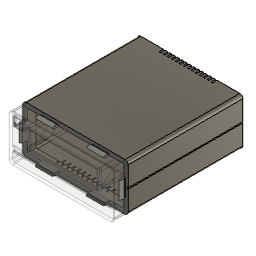
AmigaGotekEnclosure (Autodesk Fusion 360 design; units mm, degrees)
Autodesk Fusion 360 part; units mm, degrees
note: some values were not read from the file. Chosen so that the rebuilt part matches the saved one: which bodies a step acts on; which face or edge a step refers to.
(part 1 of 3)
sketch "Sketch1" plane through (0, 0, 0) normal (0, 1, 0) x (1, 0, 0) in component "face"
  line L0 (77.7875, 34.925) -> (-77.7875, 34.925)
  line L1 (-77.7875, 34.925) -> (-77.7875, -34.925)
  line L2 (-77.7875, -34.925) -> (77.7875, -34.925)
  line L3 (77.7875, -34.925) -> (77.7875, 34.925)
  line L4 (77.7875, 34.925) -> (-77.7875, -34.925) construction
  line L5 (-77.7875, 34.925) -> (77.7875, -34.925) construction
  dimension "d29" = 155.575
  dimension "d30" = 69.85
  constraint horizontal L0
  constraint perpendicular L0 L1
  constraint parallel L0 L2
  constraint parallel L1 L3
  constraint coincident L4 origin
  constraint coincident L5 origin
  measures "d29" distance of L1.end L2.end
  measures "d30" distance of L0.end L1.end
extrude "Extrude1" add sketch "Sketch1" against normal blind 19.05 draft -1 makes body 1 in component "face"
fillet "Fillet1" radius 4.572 4 edges at (-77.621241, -9.525, 34.758741) (77.621241, -9.525, 34.758741) (77.621241, -9.525, -34.758741) (-77.621241, -9.525, -34.758741) on bodies 1 in component "face"
shell "Shell1" thickness 2.38125 removed faces 1 at (-24.405399, 0, -11.641667) on bodies 1 in component "face"
sketch "Sketch2" plane through (0, -19.05, 0) normal (0, -1, 0) x (1, 0, 0) in component "face"
  ellipse E0 centre (-72.882285, -30.019785) end of major axis (-76.116162, -33.253662) minor radius 4.572 (-77.454981, -30.021177) -> (-72.883677, -34.592481) ccw
  line L0 (-72.883677, -34.592481) -> (72.883677, -34.592481)
  ellipse E1 centre (72.882285, -30.019785) end of major axis (76.116162, -33.253662) minor radius 4.572 (72.883677, -34.592481) -> (77.454981, -30.021177) ccw
  line L1 (77.454981, -30.021177) -> (77.454981, 30.021177)
  ellipse E2 centre (72.882285, 30.019785) end of major axis (76.116162, 33.253662) minor radius 4.572 (77.454981, 30.021177) -> (72.883677, 34.592481) ccw
  line L2 (72.883677, 34.592481) -> (-72.883677, 34.592481)
  ellipse E3 centre (-72.882285, 30.019785) end of major axis (-76.116162, 33.253662) minor radius 4.572 (-72.883677, 34.592481) -> (-77.454981, 30.021177) ccw
  line L3 (-77.454981, 30.021177) -> (-77.454981, -30.021177)
  line L4 (71.4375, -17.526856) -> (-71.4375, -17.526856)
  line L5 (-71.4375, -17.526856) -> (-71.4375, -15.145606)
  line L6 (-71.4375, -15.145606) -> (71.4375, -15.145606)
  line L7 (71.4375, -15.145606) -> (71.4375, -17.526856)
  line L8 (71.4375, -17.526856) -> (-71.4375, -15.145606) construction
  line L9 (-71.4375, -17.526856) -> (71.4375, -15.145606) construction
  line L10 (6.221758, -34.592481) -> (6.221758, -17.526856) construction
  point P0 (0, -16.336231)
  dimension "d36" = 142.875
  dimension "d37" = 2.38125
  dimension "d38" = 17.065625
  constraint horizontal L4
  constraint perpendicular L4 L5
  constraint parallel L4 L6
  constraint parallel L5 L7
  constraint perpendicular L4 L10
extrude "Extrude2" cut sketch "Sketch2" against normal up to surface (2.38125 mm away) contours L4 L5 L6 L7 picked at (-23.8125, -15.939356) bodies 1 in component "face"
sketch "Sketch3" plane through (0, -16.66875, 0) normal (0, 1, 0) x (-1, 0, 0) in component "face"
  line L0 (-71.4375, -17.526856) -> (-71.4375, -15.145606)
  line L1 (-71.4375, -15.145606) -> (71.4375, -15.145606)
  line L2 (71.4375, -15.145606) -> (71.4375, -17.526856)
  line L3 (71.4375, -17.526856) -> (-71.4375, -17.526856)
  ellipse E0 centre (72.923849, -30.061349) end of major axis (74.473416, -31.610916) minor radius 2.19075 (72.924517, -32.252433) -> (75.114933, -30.062017) ccw
  line L4 (75.114933, -30.062017) -> (75.114933, 30.062017)
  ellipse E1 centre (72.923849, 30.061349) end of major axis (74.473416, 31.610916) minor radius 2.19075 (75.114933, 30.062017) -> (72.924517, 32.252433) ccw
  line L5 (72.924517, 32.252433) -> (-72.924517, 32.252433)
  ellipse E2 centre (-72.923849, 30.061349) end of major axis (-74.473416, 31.610916) minor radius 2.19075 (-72.924517, 32.252433) -> (-75.114933, 30.062017) ccw
  line L6 (-75.114933, 30.062017) -> (-75.114933, -30.062017)
  ellipse E3 centre (-72.923849, -30.061349) end of major axis (-74.473416, -31.610916) minor radius 2.19075 (-75.114933, -30.062017) -> (-72.924517, -32.252433) ccw
  line L7 (-72.924517, -32.252433) -> (72.924517, -32.252433)
  line L8 (0, -15.145606) -> (0, 32.252433) construction
  line L9 (53.43525, -6.329399) -> (-53.43525, -6.329399)
  line L10 (-53.43525, -6.329399) -> (-53.43525, 23.436226)
  line L11 (-53.43525, 23.436226) -> (53.43525, 23.436226)
  line L12 (53.43525, 23.436226) -> (53.43525, -6.329399)
  line L13 (53.43525, -6.329399) -> (-53.43525, 23.436226) construction
  line L14 (-53.43525, -6.329399) -> (53.43525, 23.436226) construction
  point P0 (0, 8.553414)
  dimension "d42" = 106.8705
  dimension "d43" = 29.765625
  constraint horizontal L9
  constraint perpendicular L9 L10
  constraint parallel L9 L11
  constraint parallel L10 L12
extrude "Extrude3" add sketch "Sketch3" along normal blind 38.1 contours L9 L10 L11 L12 picked at (17.81175, 13.514351) bodies 1 in component "face"
shell "Shell2" thickness 2.38125 removed faces 1 at (-17.81175, 21.43125, 13.514351) on bodies 1 in component "face"
ref_plane "WorkPlane4" through (53.43525, 2.38125, 8.553414) normal (1, 0, 0) x (0, 0, -1) in component "face"
sketch "Sketch8" plane through (53.43525, 0, 0) normal (1, 0, 0) x (0, 1, 0) in component "face"
  line L0 (-16.66875, 23.436226) -> (-16.66875, -6.329399)
  line L1 (-16.66875, -6.329399) -> (-16.66875, 23.436226)
  line L2 (-16.66875, -17.526856) -> (-16.66875, -15.145606)
  line L3 (-16.66875, -15.145606) -> (-16.66875, -17.526856)
  line L4 (-16.66875, -32.252433) -> (-16.66875, -30.062017)
  line L5 (-16.66875, -30.062017) -> (-16.66875, 30.062017)
  line L6 (-16.66875, 30.062017) -> (-16.66875, 32.252433)
  line L7 (-16.66875, 30.062017) -> (-16.66875, 32.252433)
  line L8 (-16.66875, 30.062017) -> (-16.66875, -30.062017)
  line L9 (-16.66875, -32.252433) -> (-16.66875, -30.062017)
  line L10 (-16.66875, -3.948149) -> (21.43125, -3.948149)
  line L11 (21.43125, -3.948149) -> (-16.66875, -3.948149)
  line L12 (-16.66875, 21.054976) -> (21.43125, 21.054976)
  line L13 (21.43125, 21.054976) -> (-16.66875, 21.054976)
  line L14 (-16.66875, 21.054976) -> (-13.890625, 21.054976)
  line L15 (-13.890625, 21.054976) -> (-13.890625, -3.948149)
  line L16 (-13.890625, -3.948149) -> (-16.66875, -3.948149)
  line L17 (-16.66875, -3.948149) -> (-16.66875, 21.054976)
  dimension "d60" = 2.778125
  constraint horizontal L14
  constraint vertical L15
  constraint horizontal L16
  constraint vertical L17
extrude "Extrude6" cut sketch "Sketch8" against normal up to surface (106.8705 mm away) bodies 1 in component "face"
ref_plane "WorkPlane5" through (0, 2.38125, -3.948149) normal (0, 0, 1) x (1, 0, 0) in component "face"
sketch "Sketch9" plane through (0, 0, -3.948149) normal (0, 0, 1) x (1, 0, 0) in component "face"
  line L0 (-51.054, -13.890625) -> (-51.054, 21.43125) construction
  line L1 (-51.054, 21.43125) -> (-51.054, -13.890625) construction
  line L2 (51.054, -13.890625) -> (51.054, 21.43125) construction
  line L3 (51.054, 21.43125) -> (51.054, -13.890625) construction
  line L4 (-51.054, -13.890625) -> (51.054, -13.890625) construction
  line L5 (0, -13.890625) -> (0, 16.544917) construction
  line L6 (-51.054, -13.890625) -> (-49.863375, -13.890625)
  line L7 (-49.863375, -13.890625) -> (-51.054, 21.43125)
  line L8 (-51.054, 21.43125) -> (-51.054, -13.890625)
  line L9 (51.054, -13.890625) -> (49.863375, -13.890625)
  line L10 (49.863375, -13.890625) -> (51.054, 21.43125)
  line L11 (51.054, 21.43125) -> (51.054, -13.890625)
  dimension "d64" = 1.190625
  constraint perpendicular L4 L5
  constraint perpendicular L0 L6
extrude "Extrude7" add sketch "Sketch9" along normal up to surface (25.003125 mm away) bodies 1 in component "face"
ref_plane "WorkPlane6" through (-51.649313, -13.890625, 8.553414) normal (0, -1, 0) x (0, 0, 1) in component "face"
sketch "Sketch10" plane through (0, -13.890625, 0) normal (0, -1, 0) x (-1, 0, 0) in component "face"
  line L0 (51.054, -21.054976) -> (49.863375, -21.054976)
  line L1 (49.863375, -21.054976) -> (49.863375, 3.948149)
  line L2 (49.863375, 3.948149) -> (51.054, 3.948149)
  line L3 (51.054, 3.948149) -> (51.054, -21.054976)
  line L4 (-49.863375, -21.054976) -> (-51.054, -21.054976)
  line L5 (-51.054, -21.054976) -> (-51.054, 3.948149)
  line L6 (-51.054, 3.948149) -> (-49.863375, 3.948149)
  line L7 (-49.863375, 3.948149) -> (-49.863375, -21.054976)
  line L8 (51.054, 3.948149) -> (49.863375, 3.948149)
  line L9 (49.863375, 3.948149) -> (53.43525, 3.948149)
  line L10 (53.43525, 3.948149) -> (-53.43525, 3.948149)
  line L11 (-53.43525, 3.948149) -> (-49.863375, 3.948149)
  line L12 (-49.863375, 3.948149) -> (-51.054, 3.948149)
  line L13 (-51.054, 3.948149) -> (51.054, 3.948149)
  line L14 (49.863375, -21.054976) -> (51.054, -21.054976)
  line L15 (51.054, -21.054976) -> (-51.054, -21.054976)
  line L16 (-51.054, -21.054976) -> (-49.863375, -21.054976)
  line L17 (-49.863375, -21.054976) -> (-53.43525, -21.054976)
  line L18 (-53.43525, -21.054976) -> (53.43525, -21.054976)
  line L19 (53.43525, -21.054976) -> (49.863375, -21.054976)
  line L20 (53.43525, 3.948149) -> (53.43525, -21.054976)
  line L21 (53.43525, -21.054976) -> (53.43525, -23.436226)
  line L22 (53.43525, -23.436226) -> (53.43525, 6.329399)
  line L23 (53.43525, 6.329399) -> (53.43525, 3.948149)
  line L24 (-53.43525, -21.054976) -> (-53.43525, 3.948149)
  line L25 (-53.43525, 3.948149) -> (-53.43525, 6.329399)
  line L26 (-53.43525, 6.329399) -> (-53.43525, -23.436226)
  line L27 (-53.43525, -23.436226) -> (-53.43525, -21.054976)
  line L28 (49.863375, 3.948149) -> (-49.863375, 3.948149) construction
  line L29 (0, 3.948149) -> (0, -21.054976) construction
  line L30 (51.054, 3.948149) -> (51.054, -15.498726) construction
  line L31 (51.054, -15.498726) -> (49.863375, 3.948149)
  line L32 (49.863375, 3.948149) -> (49.863375, -21.054976)
  line L33 (49.863375, -21.054976) -> (51.054, -21.054976)
  line L34 (51.054, -21.054976) -> (51.054, -15.498726)
  line L35 (-49.863375, -21.054976) -> (-51.054, -21.054976)
  line L36 (-49.863375, 3.948149) -> (-49.863375, -21.054976)
  line L37 (-51.054, -21.054976) -> (-51.054, -15.498726)
  line L38 (-51.054, -15.498726) -> (-49.863375, 3.948149)
  dimension "d68" = 19.446875
  constraint perpendicular L8 L30
extrude "Extrude8" cut sketch "Sketch10" against normal up to surface (35.321875 mm away) contours L0 L1 L3 L14 L15 L18 L19 L31 L32 L33 L34 | L4 L5 L7 L15 L16 L17 L18 L35 L36 L37 L38 picked at (50.26025, -10.868518) picked at (-50.26025, -10.868518) bodies 1 in component "face"
sketch "Sketch11" plane through (53.43525, 0, 0) normal (1, 0, 0) x (0, 1, 0) in component "face"
  line L0 (-16.66875, 21.054976) -> (-13.890625, 21.054976)
  line L1 (-13.890625, 21.054976) -> (-13.890625, -3.948149)
  line L2 (-13.890625, -3.948149) -> (-16.66875, -3.948149)
  line L3 (-16.66875, -3.948149) -> (-16.66875, -6.329399)
  line L4 (-16.66875, -6.329399) -> (21.43125, -6.329399)
  line L5 (21.43125, -6.329399) -> (21.43125, 23.436226)
  line L6 (21.43125, 23.436226) -> (-16.66875, 23.436226)
  line L7 (-16.66875, 23.436226) -> (-16.66875, 21.054976)
  line L8 (-13.890625, -3.948149) -> (21.43125, -3.948149)
  line L9 (21.43125, -3.948149) -> (-13.890625, -3.948149)
  line L10 (-13.890625, -3.948149) -> (-16.66875, -3.948149)
  line L11 (-16.66875, -3.948149) -> (-13.890625, -3.948149)
  line L12 (-13.890625, 21.054976) -> (-13.890625, 15.498726)
  line L13 (-13.890625, 15.498726) -> (-13.890625, -3.948149)
  line L14 (-13.890625, -3.948149) -> (-13.890625, 21.054976)
  line L15 (-13.890625, -3.948149) -> (5.159375, -3.948149)
  line L16 (5.159375, -3.948149) -> (5.159375, -3.154399)
  line L17 (5.159375, -3.154399) -> (-13.890625, -3.154399)
  line L18 (-13.890625, -3.154399) -> (-13.890625, -3.948149)
  dimension "d73" = 19.05
  dimension "d74" = 0.79375
  constraint horizontal L15
  constraint vertical L16
  constraint horizontal L17
  constraint vertical L18
extrude "Extrude9" cut sketch "Sketch11" against normal up to surface (106.8705 mm away) contours L1 L8 L9 L13 L14 L15 L16 L17 L18 picked at (-7.540625, -3.683566) bodies 1 in component "face"
ref_plane "WorkPlane7" through (0, -16.66875, 0) normal (0, 1, 0) x (1, 0, 0) in component "face"
sketch "Sketch14" plane through (0, -16.66875, 0) normal (0, 1, 0) x (1, 0, 0) in component "face"
  line L0 (51.054, -21.054976) -> (51.054, -15.498726)
  line L1 (51.054, -15.498726) -> (51.054, -21.054976)
  line L2 (51.054, -21.054976) -> (53.43525, -21.054976)
  line L3 (53.43525, -21.054976) -> (-53.43525, -21.054976)
  line L4 (-53.43525, -21.054976) -> (-51.054, -21.054976)
  line L5 (-51.054, -21.054976) -> (51.054, -21.054976)
  line L6 (-51.054, -15.498726) -> (-51.054, -21.054976)
  line L7 (-51.054, -21.054976) -> (-51.054, -15.498726)
  line L8 (50.50551, 3.948149) -> (51.054, 3.948149)
  line L9 (51.054, 3.948149) -> (-51.054, 3.948149)
  line L10 (-51.054, 3.948149) -> (-50.50551, 3.948149)
  line L11 (-50.50551, 3.948149) -> (-53.43525, 3.948149)
  line L12 (-53.43525, 3.948149) -> (53.43525, 3.948149)
  line L13 (53.43525, 3.948149) -> (50.50551, 3.948149)
  line L14 (51.054, -21.054976) -> (-51.054, -21.054976) construction
  line L15 (-51.054, -21.054976) -> (-51.054, 3.948149) construction
  line L16 (-51.054, 3.948149) -> (51.054, 3.948149) construction
  line L17 (51.054, 3.948149) -> (51.054, -21.054976) construction
  line L18 (-50.26025, -20.261226) -> (-50.26025, 3.154399)
  line L19 (-50.26025, 3.154399) -> (50.26025, 3.154399)
  line L20 (50.26025, 3.154399) -> (50.26025, -20.261226)
  line L21 (50.26025, -20.261226) -> (-50.26025, -20.261226)
  dimension "d81" = 0.79375
  constraint horizontal L14
  constraint vertical L15
  constraint horizontal L16
  constraint vertical L17
extrude "Extrude10" cut sketch "Sketch14" against normal up to surface (2.38125 mm away) bodies 1 in component "face"
ref_plane "WorkPlane8" through (0, 0, 0) normal (1, 0, 0) x (0, 1, 0) in component "face"
sketch "Sketch15" plane through (0, 0, 0) normal (1, 0, 0) x (0, 1, 0) in component "face"
  line L0 (-19.05, -3.154399) -> (-16.66875, -3.154399)
  line L1 (-16.66875, -3.154399) -> (-19.05, -3.154399)
  line L2 (-16.66875, 20.261226) -> (-16.66875, -3.154399)
  line L3 (-16.66875, -3.154399) -> (-16.66875, 20.261226)
  line L4 (-16.66875, -3.948149) -> (-16.66875, -6.329399)
  line L5 (-16.66875, -6.329399) -> (-16.66875, -3.948149)
  line L6 (-16.66875, -32.252433) -> (-16.66875, -30.062017)
  line L7 (-16.66875, -30.062017) -> (-16.66875, 30.062017)
  line L8 (-16.66875, 30.062017) -> (-16.66875, 32.252433)
  line L9 (-16.66875, 30.062017) -> (-16.66875, 32.252433)
  line L10 (-16.66875, 30.062017) -> (-16.66875, -30.062017)
  line L11 (-16.66875, -32.252433) -> (-16.66875, -30.062017)
  line L12 (-16.66875, -17.526856) -> (-16.66875, -15.145606)
  line L13 (-16.66875, -15.145606) -> (-16.66875, -17.526856)
  line L14 (-16.66875, 21.054976) -> (-16.66875, 23.436226)
  line L15 (-16.66875, 23.436226) -> (-16.66875, 21.054976)
  line L16 (-16.66875, -3.154399) -> (-19.05, -3.154399)
  line L17 (-19.05, -3.154399) -> (-19.05, -5.535649)
  line L18 (-19.05, -5.535649) -> (-16.66875, -3.154399)
  constraint perpendicular L1 L17
  constraint equal L16 L17
sweep "Sweep1" cut profiles "Sketch15" along 4 edges at (0, -16.66875, 20.261226) (-50.26025, -16.66875, 8.553414) (0, -16.66875, -3.154399) (50.26025, -16.66875, 8.553414) section 1 on bodies 1 bodies 1 in component "face"
sketch "Sketch16" plane through (0, 0, 0) normal (0, 1, 0) x (-1, 0, 0) in component "face"
  ellipse E0 centre (73.214804, -30.352304) end of major axis (74.76437, -31.90187) minor radius 2.19075 (73.215471, -32.543387) -> (75.405887, -30.352971) ccw
  line L0 (73.215471, -32.543387) -> (-73.215471, -32.543387)
  ellipse E1 centre (-73.214804, -30.352304) end of major axis (-74.76437, -31.90187) minor radius 2.19075 (-75.405887, -30.352971) -> (-73.215471, -32.543387) ccw
  line L1 (-75.405887, -30.352971) -> (-75.405887, 30.352971)
  ellipse E2 centre (-73.214804, 30.352304) end of major axis (-74.76437, 31.90187) minor radius 2.19075 (-73.215471, 32.543387) -> (-75.405887, 30.352971) ccw
  line L2 (-73.215471, 32.543387) -> (73.215471, 32.543387)
  ellipse E3 centre (73.214804, 30.352304) end of major axis (74.76437, 31.90187) minor radius 2.19075 (75.405887, 30.352971) -> (73.215471, 32.543387) ccw
  line L3 (75.405887, 30.352971) -> (75.405887, -30.352971)
  ellipse E4 centre (73.214804, -30.352304) end of major axis (76.448681, -33.586181) minor radius 4.572 (73.216196, -34.925) -> (77.7875, -30.353696) ccw
  line L4 (77.7875, -30.353696) -> (77.7875, 30.353696)
  ellipse E5 centre (73.214804, 30.352304) end of major axis (76.448681, 33.586181) minor radius 4.572 (77.7875, 30.353696) -> (73.216196, 34.925) ccw
  line L5 (73.216196, 34.925) -> (-73.216196, 34.925)
  ellipse E6 centre (-73.214804, 30.352304) end of major axis (-76.448681, 33.586181) minor radius 4.572 (-73.216196, 34.925) -> (-77.7875, 30.353696) ccw
  line L6 (-77.7875, 30.353696) -> (-77.7875, -30.353696)
  ellipse E7 centre (-73.214804, -30.352304) end of major axis (-76.448681, -33.586181) minor radius 4.572 (-77.7875, -30.353696) -> (-73.216196, -34.925) ccw
  line L7 (-73.216196, -34.925) -> (73.216196, -34.925)
  line L8 (-77.7875, 30.353696) -> (-77.7875, -30.353696)
  ellipse E8 centre (-73.214804, 30.352304) end of major axis (-76.448681, 33.586181) minor radius 4.572 (-73.216196, 34.925) -> (-77.7875, 30.353696) ccw
  line L9 (73.216196, 34.925) -> (-73.216196, 34.925)
  ellipse E9 centre (-73.214804, -30.352304) end of major axis (-76.448681, -33.586181) minor radius 4.572 (-77.7875, -30.353696) -> (-73.216196, -34.925) ccw
  line L10 (-73.216196, -34.925) -> (73.216196, -34.925)
  ellipse E10 centre (73.214804, -30.352304) end of major axis (76.448681, -33.586181) minor radius 4.572 (73.216196, -34.925) -> (77.7875, -30.353696) ccw
  line L11 (77.7875, -30.353696) -> (77.7875, 30.353696)
  ellipse E11 centre (73.214804, 30.352304) end of major axis (76.448681, 33.586181) minor radius 4.572 (77.7875, 30.353696) -> (73.216196, 34.925) ccw
  line L12 (-73.216196, -33.3375) -> (73.216196, -33.3375)
  spline S0 degree 3 poles (73.216196, -33.3375) (74.237846, -33.3375) (75.241029, -32.771776) (75.769487, -31.897837) (76.049372, -31.434976) (76.2, -30.894788) (76.2, -30.353696) knots -0.78524587 -0.78524587 -0.78524587 -0.78524587 0.2414707 0.2414707 0.2414707 0.78524587 0.78524587 0.78524587 0.78524587
  line L13 (76.2, -30.353696) -> (76.2, 30.353696)
  spline S1 degree 3 poles (76.2, 30.353696) (76.2, 31.375346) (75.634276, 32.378529) (74.760337, 32.906987) (74.297476, 33.186872) (73.757288, 33.3375) (73.216196, 33.3375) knots -0.78524587 -0.78524587 -0.78524587 -0.78524587 0.2414707 0.2414707 0.2414707 0.78524587 0.78524587 0.78524587 0.78524587
  line L14 (73.216196, 33.3375) -> (-73.216196, 33.3375)
  spline S2 degree 3 poles (-73.216196, 33.3375) (-74.237846, 33.3375) (-75.241029, 32.771776) (-75.769487, 31.897837) (-76.049372, 31.434976) (-76.2, 30.894788) (-76.2, 30.353696) knots -0.78524587 -0.78524587 -0.78524587 -0.78524587 0.2414707 0.2414707 0.2414707 0.78524587 0.78524587 0.78524587 0.78524587
  line L15 (-76.2, 30.353696) -> (-76.2, -30.353696)
  spline S3 degree 3 poles (-76.2, -30.353696) (-76.2, -31.375346) (-75.634276, -32.378529) (-74.760337, -32.906987) (-74.297476, -33.186872) (-73.757288, -33.3375) (-73.216196, -33.3375) knots -0.78524587 -0.78524587 -0.78524587 -0.78524587 0.2414707 0.2414707 0.2414707 0.78524587 0.78524587 0.78524587 0.78524587
  line L16 (-73.216196, -30.95625) -> (73.216196, -30.95625)
  spline S4 degree 3 poles (73.216196, -30.95625) (73.53236, -30.95625) (73.81875, -30.66986) (73.81875, -30.353696) knots -0.78524587 -0.78524587 -0.78524587 -0.78524587 0.78524587 0.78524587 0.78524587 0.78524587
  line L17 (73.81875, -30.353696) -> (73.81875, 30.353696)
  spline S5 degree 3 poles (73.81875, 30.353696) (73.81875, 30.66986) (73.53236, 30.95625) (73.216196, 30.95625) knots -0.78524587 -0.78524587 -0.78524587 -0.78524587 0.78524587 0.78524587 0.78524587 0.78524587
  line L18 (73.216196, 30.95625) -> (-73.216196, 30.95625)
  spline S6 degree 3 poles (-73.216196, 30.95625) (-73.53236, 30.95625) (-73.81875, 30.66986) (-73.81875, 30.353696) knots -0.78524587 -0.78524587 -0.78524587 -0.78524587 0.78524587 0.78524587 0.78524587 0.78524587
  line L19 (-73.81875, 30.353696) -> (-73.81875, -30.353696)
  spline S7 degree 3 poles (-73.81875, -30.353696) (-73.81875, -30.66986) (-73.53236, -30.95625) (-73.216196, -30.95625) knots -0.78524587 -0.78524587 -0.78524587 -0.78524587 0.78524587 0.78524587 0.78524587 0.78524587
extrude "Extrude12" add sketch "Sketch16" along normal blind 1.5875 contours E0 L0 E1 L1 E2 L2 E3 L3 | L12 S0 L13 S1 L14 S2 L15 S3 picked at (-24.405157, -31.485296) picked at (24.405157, -33.072796) bodies 1 in component "face"
sketch "Sketch17" plane through (53.43525, 0, 0) normal (1, 0, 0) x (0, 1, 0) in component "face"
  line L0 (0, -30.95625) -> (0, -30.353696)
  line L1 (0, -30.353696) -> (0, -30.95625)
  line L2 (0, -30.353696) -> (0, 30.353696)
  line L3 (0, 30.95625) -> (0, 30.353696)
  line L4 (0, 30.353696) -> (0, 30.95625)
  line L5 (0, 30.353696) -> (0, -30.353696)
  line L6 (0, -30.352971) -> (0, -32.543387)
  line L7 (0, -30.352971) -> (0, -32.543387)
  line L8 (0, -30.352971) -> (0, 30.352971)
  line L9 (0, 32.543387) -> (0, 30.352971)
  line L10 (0, 32.543387) -> (0, 30.352971)
  line L11 (0, 30.352971) -> (0, -30.352971)
  line L12 (0, -32.543387) -> (-16.66875, -32.252433)
  line L13 (-16.66875, -32.252433) -> (0, -32.543387)
  line L14 (0, -30.95625) -> (0, -32.543387)
  line L15 (0, -32.543387) -> (-1.586896, -32.515688)
  line L16 (0, -30.95625) -> (-1.586896, -32.515688)
  constraint parallel L13 L15
  constraint equal L14 L15
sweep "Sweep2" add profiles "Sketch17" along 8 edges at (75.405887, 0, 0) (74.76437, 0, 31.90187) (0, 0, 32.543387) (-74.76437, 0, 31.90187) (-75.405887, 0, 0) (-74.76437, 0, -31.90187) (0, 0, -32.543387) (74.76437, 0, -31.90187) section 1 on bodies 1 bodies 1 in component "face"
sketch "Sketch2 (2)" plane through (0, 1.5875, 0) normal (0, 1, 0) x (-1, 0, 0) in component "enclosure"
  spline S0 degree 3 poles (-73.216196, -30.95625) (-73.53236, -30.95625) (-73.81875, -30.66986) (-73.81875, -30.353696) knots -0.78524587 -0.78524587 -0.78524587 -0.78524587 0.78524587 0.78524587 0.78524587 0.78524587
  line L0 (-73.81875, -30.353696) -> (-73.81875, 30.353696)
  spline S1 degree 3 poles (-73.81875, 30.353696) (-73.81875, 30.66986) (-73.53236, 30.95625) (-73.216196, 30.95625) knots -0.78524587 -0.78524587 -0.78524587 -0.78524587 0.78524587 0.78524587 0.78524587 0.78524587
  line L1 (-73.216196, 30.95625) -> (73.216196, 30.95625)
  spline S2 degree 3 poles (73.216196, 30.95625) (73.53236, 30.95625) (73.81875, 30.66986) (73.81875, 30.353696) knots -0.78524587 -0.78524587 -0.78524587 -0.78524587 0.78524587 0.78524587 0.78524587 0.78524587
  line L2 (73.81875, 30.353696) -> (73.81875, -30.353696)
  spline S3 degree 3 poles (73.81875, -30.353696) (73.81875, -30.66986) (73.53236, -30.95625) (73.216196, -30.95625) knots -0.78524587 -0.78524587 -0.78524587 -0.78524587 0.78524587 0.78524587 0.78524587 0.78524587
  line L3 (73.216196, -30.95625) -> (-73.216196, -30.95625)
  spline S4 degree 3 poles (-76.2, -30.353696) (-76.2, -31.375346) (-75.634276, -32.378529) (-74.760337, -32.906987) (-74.297476, -33.186872) (-73.757288, -33.3375) (-73.216196, -33.3375) knots -0.78524587 -0.78524587 -0.78524587 -0.78524587 0.2414707 0.2414707 0.2414707 0.78524587 0.78524587 0.78524587 0.78524587
  line L4 (-73.216196, -33.3375) -> (73.216196, -33.3375)
  spline S5 degree 3 poles (73.216196, -33.3375) (74.237846, -33.3375) (75.241029, -32.771776) (75.769487, -31.897837) (76.049372, -31.434976) (76.2, -30.894788) (76.2, -30.353696) knots -0.78524587 -0.78524587 -0.78524587 -0.78524587 0.2414707 0.2414707 0.2414707 0.78524587 0.78524587 0.78524587 0.78524587
  line L5 (76.2, -30.353696) -> (76.2, 30.353696)
  spline S6 degree 3 poles (76.2, 30.353696) (76.2, 31.375346) (75.634276, 32.378529) (74.760337, 32.906987) (74.297476, 33.186872) (73.757288, 33.3375) (73.216196, 33.3375) knots -0.78524587 -0.78524587 -0.78524587 -0.78524587 0.2414707 0.2414707 0.2414707 0.78524587 0.78524587 0.78524587 0.78524587
  line L6 (73.216196, 33.3375) -> (-73.216196, 33.3375)
  spline S7 degree 3 poles (-73.216196, 33.3375) (-74.237846, 33.3375) (-75.241029, 32.771776) (-75.769487, 31.897837) (-76.049372, 31.434976) (-76.2, 30.894788) (-76.2, 30.353696) knots -0.78524587 -0.78524587 -0.78524587 -0.78524587 0.2414707 0.2414707 0.2414707 0.78524587 0.78524587 0.78524587 0.78524587
  line L7 (-76.2, 30.353696) -> (-76.2, -30.353696)
  line L8 (-76.2, 30.353696) -> (-76.2, -30.353696)
  spline S8 degree 3 poles (-76.2, -30.353696) (-76.2, -31.375346) (-75.634276, -32.378529) (-74.760337, -32.906987) (-74.297476, -33.186872) (-73.757288, -33.3375) (-73.216196, -33.3375) knots -0.78524587 -0.78524587 -0.78524587 -0.78524587 0.2414707 0.2414707 0.2414707 0.78524587 0.78524587 0.78524587 0.78524587
  line L9 (-73.216196, -33.3375) -> (73.216196, -33.3375)
  spline S9 degree 3 poles (-73.216196, 33.3375) (-74.237846, 33.3375) (-75.241029, 32.771776) (-75.769487, 31.897837) (-76.049372, 31.434976) (-76.2, 30.894788) (-76.2, 30.353696) knots -0.78524587 -0.78524587 -0.78524587 -0.78524587 0.2414707 0.2414707 0.2414707 0.78524587 0.78524587 0.78524587 0.78524587
  line L10 (73.216196, 33.3375) -> (-73.216196, 33.3375)
  spline S10 degree 3 poles (73.216196, -33.3375) (74.237846, -33.3375) (75.241029, -32.771776) (75.769487, -31.897837) (76.049372, -31.434976) (76.2, -30.894788) (76.2, -30.353696) knots -0.78524587 -0.78524587 -0.78524587 -0.78524587 0.2414707 0.2414707 0.2414707 0.78524587 0.78524587 0.78524587 0.78524587
  line L11 (76.2, -30.353696) -> (76.2, 30.353696)
  spline S11 degree 3 poles (76.2, 30.353696) (76.2, 31.375346) (75.634276, 32.378529) (74.760337, 32.906987) (74.297476, 33.186872) (73.757288, 33.3375) (73.216196, 33.3375) knots -0.78524587 -0.78524587 -0.78524587 -0.78524587 0.2414707 0.2414707 0.2414707 0.78524587 0.78524587 0.78524587 0.78524587
  line L12 (-73.81875, -30.353696) -> (-73.81875, 30.353696)
  spline S12 degree 3 poles (-73.216196, -30.95625) (-73.53236, -30.95625) (-73.81875, -30.66986) (-73.81875, -30.353696) knots -0.78524587 -0.78524587 -0.78524587 -0.78524587 0.78524587 0.78524587 0.78524587 0.78524587
  line L13 (73.216196, -30.95625) -> (-73.216196, -30.95625)
  spline S13 degree 3 poles (-73.81875, 30.353696) (-73.81875, 30.66986) (-73.53236, 30.95625) (-73.216196, 30.95625) knots -0.78524587 -0.78524587 -0.78524587 -0.78524587 0.78524587 0.78524587 0.78524587 0.78524587
  line L14 (-73.216196, 30.95625) -> (73.216196, 30.95625)
  spline S14 degree 3 poles (73.216196, 30.95625) (73.53236, 30.95625) (73.81875, 30.66986) (73.81875, 30.353696) knots -0.78524587 -0.78524587 -0.78524587 -0.78524587 0.78524587 0.78524587 0.78524587 0.78524587
  line L15 (73.81875, 30.353696) -> (73.81875, -30.353696)
  spline S15 degree 3 poles (73.81875, -30.353696) (73.81875, -30.66986) (73.53236, -30.95625) (73.216196, -30.95625) knots -0.78524587 -0.78524587 -0.78524587 -0.78524587 0.78524587 0.78524587 0.78524587 0.78524587
  line L16 (-71.4375, 28.575) -> (71.4375, 28.575)
  line L17 (71.4375, 28.575) -> (71.4375, -28.575)
  line L18 (71.4375, -28.575) -> (-71.4375, -28.575)
  line L19 (-71.4375, -28.575) -> (-71.4375, 28.575)
  dimension "d117" = 2.38125
extrude "Extrude1'" add sketch "Sketch2 (2)" against normal blind 9.525 separate body contours S0 L0 S1 L1 S2 L2 S3 L3 L12 S12 L13 S13 L14 S14 L15 S15 | S4 L4 S5 L5 S6 L6 S7 L7 L8 S8 L9 S9 L10 S10 L11 S11 picked at (-23.8125, 30.1625) picked at (-24.405399, 32.54375) makes body 2 in component "enclosure"
combine "Combine1" operation cut target body 2 tool bodies 1 keep tools in component "enclosure"
sketch "Sketch5" plane through (0, -7.9375, 0) normal (0, -1, 0) x (1, 0, 0) in component "enclosure"
  line L0 (-73.076921, -32.404838) -> (73.076921, -32.404838)
  ellipse E0 centre (73.076254, -30.213754) end of major axis (74.62582, -31.76332) minor radius 2.19075 (73.076921, -32.404838) -> (75.267338, -30.214421) ccw
  line L1 (75.267338, -30.214421) -> (75.267338, 30.214421)
  ellipse E1 centre (73.076254, 30.213754) end of major axis (74.62582, 31.76332) minor radius 2.19075 (75.267338, 30.214421) -> (73.076921, 32.404838) ccw
  line L2 (73.076921, 32.404838) -> (-73.076921, 32.404838)
  ellipse E2 centre (-73.076254, 30.213754) end of major axis (-74.62582, 31.76332) minor radius 2.19075 (-73.076921, 32.404838) -> (-75.267338, 30.214421) ccw
  line L3 (-75.267338, 30.214421) -> (-75.267338, -30.214421)
  ellipse E3 centre (-73.076254, -30.213754) end of major axis (-74.62582, -31.76332) minor radius 2.19075 (-75.267338, -30.214421) -> (-73.076921, -32.404838) ccw
  line L4 (71.4375, -28.575) -> (-71.4375, -28.575)
  line L5 (-71.4375, -28.575) -> (-71.4375, 28.575)
  line L6 (-71.4375, 28.575) -> (71.4375, 28.575)
  line L7 (71.4375, 28.575) -> (71.4375, -28.575)
  line L8 (-71.4375, -28.575) -> (-71.4375, 28.575)
  line L9 (-71.4375, 28.575) -> (71.4375, 28.575)
  line L10 (71.4375, -28.575) -> (-71.4375, -28.575)
  line L11 (71.4375, 28.575) -> (71.4375, -28.575)
  line L12 (75.378188, -30.325272) -> (75.378188, 30.325272)
  spline S0 degree 3 poles (73.215471, 32.515516) (73.500225, 32.51198) (73.781581, 32.452973) (74.306005, 32.230508) (74.544035, 32.06915) (74.945111, 31.664102) (75.104227, 31.424229) (75.318554, 30.904269) (75.374573, 30.630196) (75.378016, 30.352971) knots 0 0 0 0 0.08543972 0.08543972 0.17090372 0.17090372 0.25644981 0.25644981 0.33963045 0.33963045 0.33963045 0.33963045
  line L13 (73.187772, 32.515688) -> (-73.187772, 32.515688)
  spline S1 degree 3 poles (-75.378016, 30.352971) (-75.37448, 30.637725) (-75.315473, 30.919081) (-75.093008, 31.443505) (-74.93165, 31.681535) (-74.526602, 32.082611) (-74.286729, 32.241727) (-73.766769, 32.456054) (-73.492696, 32.512073) (-73.215471, 32.515516) knots 0 0 0 0 0.08543972 0.08543972 0.17090372 0.17090372 0.25644981 0.25644981 0.33963045 0.33963045 0.33963045 0.33963045
  line L14 (-75.378188, 30.325272) -> (-75.378188, -30.325272)
  spline S2 degree 3 poles (-73.215471, -32.515516) (-73.500225, -32.51198) (-73.781581, -32.452973) (-74.306005, -32.230508) (-74.544035, -32.06915) (-74.945111, -31.664102) (-75.104227, -31.424229) (-75.318554, -30.904269) (-75.374573, -30.630196) (-75.378016, -30.352971) knots 0 0 0 0 0.08543972 0.08543972 0.17090372 0.17090372 0.25644981 0.25644981 0.33963045 0.33963045 0.33963045 0.33963045
  line L15 (-73.187772, -32.515688) -> (73.187772, -32.515688)
  spline S3 degree 3 poles (75.378016, -30.352971) (75.37448, -30.637725) (75.315473, -30.919081) (75.093008, -31.443505) (74.93165, -31.681535) (74.526602, -32.082611) (74.286729, -32.241727) (73.766769, -32.456054) (73.492696, -32.512073) (73.215471, -32.515516) knots 0 0 0 0 0.08543972 0.08543972 0.17090372 0.17090372 0.25644981 0.25644981 0.33963045 0.33963045 0.33963045 0.33963045
  line L16 (0, 0) -> (0, 28.575) construction
  line L17 (0, 0) -> (71.4375, 0) construction
  line L18 (71.4375, 12.7) -> (75.378016, 12.7)
  line L19 (75.378016, 12.7) -> (75.378016, -12.7)
  line L20 (75.378016, -12.7) -> (71.4375, -12.7)
  line L21 (71.4375, -12.7) -> (71.4375, 12.7)
  line L22 (75.378016, 30.352971) -> (75.378016, -30.352971) construction
  line L23 (75.378188, 30.325272) -> (75.378188, 43.581257) construction
  line L24 (73.215471, 32.515516) -> (77.094391, 32.515516) construction
  line L25 (75.378188, 32.515516) -> (0, 32.515688) construction
  line L26 (24.989094, 32.515602) -> (50.389094, 32.515602)
  line L27 (50.389094, 32.515602) -> (50.389094, 28.575)
  line L28 (50.389094, 28.575) -> (24.989094, 28.575)
  line L29 (24.989094, 28.575) -> (24.989094, 32.515602)
  line L30 (71.4375, 28.575) -> (0, 28.575) construction
  line L31 (-24.989094, 32.515602) -> (-50.389094, 32.515602)
  line L32 (-24.989094, 28.575) -> (-24.989094, 32.515602)
  line L33 (-50.389094, 28.575) -> (-24.989094, 28.575)
  line L34 (-50.389094, 32.515602) -> (-50.389094, 28.575)
  line L35 (-50.389094, -28.575) -> (-24.989094, -28.575)
  line L36 (-50.389094, -32.515602) -> (-50.389094, -28.575)
  line L37 (-24.989094, -32.515602) -> (-50.389094, -32.515602)
  line L38 (-24.989094, -28.575) -> (-24.989094, -32.515602)
  line L39 (50.389094, -28.575) -> (24.989094, -28.575)
  line L40 (24.989094, -28.575) -> (24.989094, -32.515602)
  line L41 (24.989094, -32.515602) -> (50.389094, -32.515602)
  line L42 (50.389094, -32.515602) -> (50.389094, -28.575)
  line L43 (-71.4375, -12.7) -> (-71.4375, 12.7)
  line L44 (-75.378016, 12.7) -> (-75.378016, -12.7)
  line L45 (-71.4375, 12.7) -> (-75.378016, 12.7)
  line L46 (-75.378016, -12.7) -> (-71.4375, -12.7)
  point P0 (71.4375, 0)
  point P1 (75.378188, 32.515516)
  point P2 (37.689094, 32.515602)
  dimension "d131" = 25.4
  dimension "d132" = 25.4
  constraint coincident L16.start L17.start
  constraint midpoint L6 L16.end
  constraint midpoint L7 P0
  constraint coincident P0 L17.end
  constraint horizontal L18
  constraint vertical L19
  constraint horizontal L20
  constraint vertical L21
  constraint midpoint P0 L21
  constraint collinear L19 L22
  constraint parallel L22 L23
  constraint parallel L13 L24
  constraint horizontal L26
  constraint vertical L27
  constraint horizontal L28
  constraint vertical L29
  constraint coincident L6.end L7.start
  constraint collinear L28 L30
  constraint symmetric L16 L18.start L43.end
  constraint symmetric L16 L20.end L43.start
extrude "Extrude4" cut sketch "Sketch5" against normal up to surface (9.525 mm away) contours L0 L3 E3 L4 L5 L8 L10 L36 L46 | L0 L4 L10 L38 L40 | L2 E2 L3 L5 L6 L8 L9 L34 L45 | L0 E0 L1 L4 L7 L10 L11 L20 L42 | L2 L6 L9 L29 L32 | L1 E1 L2 L6 L7 L9 L11 L18 L27 picked at (-64.967838, -31.128225) picked at (8.329698, -29.851613) picked at (-64.967838, 31.128225) picked at (64.967838, -31.128225) picked at (8.329698, 29.851613) picked at (64.967838, 31.128225) bodies 2 in component "enclosure"
sketch "Sketch6" plane through (0, 1.5875, 0) normal (0, 1, 0) x (-1, 0, 0) in component "enclosure"
  line L0 (-50.389094, 30.95625) -> (-50.389094, 28.575)
  line L1 (-50.389094, 28.575) -> (-24.989094, 28.575)
  line L2 (-24.989094, 28.575) -> (-24.989094, 30.95625)
  line L3 (-24.989094, 30.95625) -> (-50.389094, 30.95625)
  line L4 (71.4375, 12.7) -> (75.267338, 12.7)
  line L5 (50.389094, 32.404838) -> (50.389094, 28.575)
  line L6 (24.989094, 28.575) -> (24.989094, 32.404838)
  line L7 (-24.989094, 32.404838) -> (-24.989094, 28.575)
  line L8 (-50.389094, 28.575) -> (-50.389094, 32.404838)
  line L9 (-75.267338, 12.7) -> (-71.4375, 12.7)
  line L10 (-71.4375, -12.7) -> (-75.267338, -12.7)
  line L11 (-50.389094, -32.404838) -> (-50.389094, -28.575)
  line L12 (-24.989094, -28.575) -> (-24.989094, -32.404838)
  line L13 (24.989094, -32.404838) -> (24.989094, -28.575)
  line L14 (50.389094, -28.575) -> (50.389094, -32.404838)
  line L15 (75.267338, -12.7) -> (71.4375, -12.7)
  line L16 (-75.267338, 12.7) -> (75.267338, 12.7) construction
  line L17 (75.267338, -12.7) -> (-75.267338, -12.7) construction
  line L18 (-50.389094, 32.404838) -> (-50.389094, -32.404838) construction
  line L19 (-24.989094, -32.404838) -> (-24.989094, 32.404838) construction
  line L20 (24.989094, 32.404838) -> (24.989094, -32.404838) construction
  line L21 (50.389094, -32.404838) -> (50.389094, 32.404838) construction
  line L22 (0, 0) -> (0, 44.450001) construction
  line L23 (0, 0) -> (76.200002, 0) construction
  line L24 (-50.389094, 12.7) -> (-83.820003, 12.7)
  line L25 (-83.820003, 12.7) -> (-83.820003, 38.100001)
  line L26 (-83.820003, 38.100001) -> (-50.389094, 38.100001)
  line L27 (-50.389094, 38.100001) -> (-50.389094, 12.7)
  line L28 (50.389094, 12.7) -> (83.820003, 12.7)
  line L29 (83.820003, 12.7) -> (83.820003, 38.100001)
  line L30 (83.820003, 38.100001) -> (50.389094, 38.100001)
  line L31 (50.389094, 38.100001) -> (50.389094, 12.7)
  line L32 (-83.820003, -12.7) -> (-83.820003, -38.100001)
  line L33 (-50.389094, -12.7) -> (-83.820003, -12.7)
  line L34 (-83.820003, -38.100001) -> (-50.389094, -38.100001)
  line L35 (-50.389094, -38.100001) -> (-50.389094, -12.7)
  line L36 (50.389094, -38.100001) -> (50.389094, -12.7)
  line L37 (50.389094, -12.7) -> (83.820003, -12.7)
  line L38 (83.820003, -12.7) -> (83.820003, -38.100001)
  line L39 (83.820003, -38.100001) -> (50.389094, -38.100001)
  line L40 (-24.989094, 12.7) -> (24.989094, 12.7)
  line L41 (24.989094, 12.7) -> (24.989094, 39.628809)
  line L42 (24.989094, 39.628809) -> (-24.989094, 39.628809)
  line L43 (-24.989094, 39.628809) -> (-24.989094, 12.7)
  line L44 (-24.989094, -39.628809) -> (-24.989094, -12.7)
  line L45 (24.989094, -39.628809) -> (-24.989094, -39.628809)
  line L46 (24.989094, -12.7) -> (24.989094, -39.628809)
  line L47 (-24.989094, -12.7) -> (24.989094, -12.7)
  constraint coincident L22.start L23.start
  constraint perpendicular L16 L22
  constraint perpendicular L21 L23
  constraint horizontal L24
  constraint vertical L25
  constraint horizontal L26
  constraint vertical L27
  constraint horizontal L40
  constraint vertical L41
  constraint horizontal L42
  constraint vertical L43
extrude "Extrude5" cut sketch "Sketch6" against normal up to surface (9.525 mm away) contours L0 L8 L9 L24 L25 L26 L27 | L2 L6 L7 L40 L41 L42 L43 | L4 L5 L28 L29 L30 L31 | L10 L11 L32 L33 L34 L35 | L12 L13 L44 L45 L46 L47 | L14 L15 L36 L37 L38 L39 picked at (-68.548866, 27.252084) picked at (-8.329698, 17.991667) picked at (68.548866, 26.458334) picked at (-68.548866, -26.458334) picked at (8.329698, -17.991667) picked at (68.548866, -26.458334) bodies 2 makes body 3 at (41.922427, -4.7625, -28.575) makes body 4 at (71.4375, -1.5875, -4.233333) makes body 5 at (-41.922427, -1.5875, -28.575) makes body 6 at (-33.455761, -1.5875, 28.575) makes body 7 at (-71.4375, -1.5875, 4.233333) in component "enclosure"
chamfer "Chamfer1" distance 2.38125 angle 45 6 edges at (37.689094, -7.9375, 28.575) (37.689094, -7.9375, -28.575) (-37.689094, -7.9375, -28.575) (-37.689094, -7.9375, 28.575) (-71.4375, -7.9375, 0) (71.4375, -7.9375, 0) on bodies 2 3 4 5 6 7 in component "enclosure"
sketch "Sketch7" plane through (0, 1.5875, 0) normal (0, 1, 0) x (-1, 0, 0) in component "enclosure"
  line L0 (-50.389094, 30.95625) -> (-50.389094, 28.575)
  line L1 (-50.389094, 28.575) -> (-24.989094, 28.575)
  line L2 (-24.989094, 28.575) -> (-24.989094, 30.95625)
  line L3 (-24.989094, 30.95625) -> (-50.389094, 30.95625)
  ellipse E0 centre (-73.214804, 30.352304) end of major axis (-76.448681, 33.586181) minor radius 4.572 (-73.216196, 34.925) -> (-77.7875, 30.353696) ccw
  line L4 (-77.7875, 30.353696) -> (-77.7875, -30.353696)
  line L5 (73.216196, 34.925) -> (-73.216196, 34.925)
  ellipse E1 centre (-73.214804, -30.352304) end of major axis (-76.448681, -33.586181) minor radius 4.572 (-77.7875, -30.353696) -> (-73.216196, -34.925) ccw
  line L6 (-73.216196, -34.925) -> (73.216196, -34.925)
  ellipse E2 centre (73.214804, 30.352304) end of major axis (76.448681, 33.586181) minor radius 4.572 (77.7875, 30.353696) -> (73.216196, 34.925) ccw
  line L7 (77.7875, -30.353696) -> (77.7875, 30.353696)
  ellipse E3 centre (73.214804, -30.352304) end of major axis (76.448681, -33.586181) minor radius 4.572 (73.216196, -34.925) -> (77.7875, -30.353696) ccw
  line L8 (71.4375, 12.7) -> (71.4375, -12.7)
  line L9 (50.389094, -28.575) -> (24.989094, -28.575)
  line L10 (-24.989094, -28.575) -> (-50.389094, -28.575)
  line L11 (24.989094, 28.575) -> (50.389094, 28.575)
  line L12 (-50.389094, 28.575) -> (-24.989094, 28.575)
  line L13 (-71.4375, -12.7) -> (-71.4375, 12.7)
  line L14 (-50.389094, 28.575) -> (86.360003, 28.575) construction
  line L15 (71.4375, -12.7) -> (71.4375, 43.180001) construction
  line L16 (50.389094, 28.575) -> (-90.691859, 28.575) construction
  line L17 (-71.4375, -12.7) -> (-71.4375, 46.842127) construction
  line L18 (-71.4375, 12.7) -> (-71.4375, -45.720001) construction
  line L19 (-50.389094, -28.575) -> (88.900003, -28.575) construction
  line L20 (71.4375, 12.7) -> (71.4375, -43.180001) construction
  line L21 (50.389094, -28.575) -> (-86.360003, -28.575) construction
  line L22 (-71.4375, 28.575) -> (71.4375, 28.575)
  line L23 (71.4375, 28.575) -> (71.4375, -28.575)
  line L24 (71.4375, -28.575) -> (-71.4375, -28.575)
  line L25 (-71.4375, -28.575) -> (-71.4375, 28.575)
  line L26 (-73.216196, 34.925) -> (91.440003, 34.925) construction
  line L27 (73.216196, 34.925) -> (-88.900003, 34.925) construction
  line L28 (-77.7875, 30.353696) -> (-77.7875, -50.800002) construction
  line L29 (-77.7875, -30.353696) -> (-77.7875, 53.340002) construction
  line L30 (73.216196, -34.925) -> (-90.353161, -34.925) construction
  line L31 (-73.216196, -34.925) -> (88.900003, -34.925) construction
  line L32 (77.7875, -30.353696) -> (77.7875, 47.143219) construction
  line L33 (77.7875, 30.353696) -> (77.7875, -45.720001) construction
  line L34 (-73.2155, 34.925) -> (73.2155, 34.925)
  line L35 (77.7875, 30.353) -> (77.7875, -30.353)
  line L36 (73.2155, -34.925) -> (-73.2155, -34.925)
  line L37 (-77.7875, -30.353) -> (-77.7875, 30.353)
  arc A0 (-73.2155, 34.925) -> (-77.7875, 30.353) centre (-73.2155, 30.353) ccw
  arc A1 (-77.7875, -30.353) -> (-73.2155, -34.925) centre (-73.2155, -30.353) ccw
  arc A2 (73.2155, -34.925) -> (77.7875, -30.353) centre (73.2155, -30.353) ccw
  arc A3 (77.7875, 30.353) -> (73.2155, 34.925) centre (73.2155, 30.353) ccw
  dimension "d138" = 4.572
  dimension "d139" = 4.572
  dimension "d140" = 4.572
  dimension "d141" = 4.572
  constraint perpendicular L7 L14
  constraint coincident L8.end L15.start
  constraint perpendicular L5 L15
  constraint perpendicular L4 L16
  constraint coincident L13.start L17.start
  constraint perpendicular L5 L17
  constraint coincident L13.end L18.start
  constraint perpendicular L6 L18
  constraint perpendicular L7 L19
  constraint coincident L8.start L20.start
  constraint perpendicular L6 L20
  constraint perpendicular L4 L21
  constraint horizontal L22
  constraint vertical L23
  constraint horizontal L24
  constraint vertical L25
  constraint coincident L20 L23.end
  constraint coincident L19 L23.end
  constraint coincident L16 L22.start
  constraint coincident L17 L22.start
  constraint tangent E0 L26
  constraint perpendicular L15 L26
  constraint tangent E2 L27
  constraint parallel L26 L27
  constraint tangent E0 L28
  constraint perpendicular L21 L28
  constraint tangent E1 L29
  constraint perpendicular L27 L29
  constraint tangent E3 L30
  constraint perpendicular L28 L30
  constraint tangent E1 L31
  constraint parallel L30 L31
  constraint tangent E3 L32
  constraint perpendicular L26 L32
  constraint tangent E2 L33
  constraint perpendicular L31 L33
  constraint horizontal L34
  constraint vertical L35
  constraint horizontal L36
  constraint vertical L37
  constraint tangent L37 A0
  constraint tangent L34 A0
  constraint tangent L37 A1
  constraint tangent L36 A1
  constraint tangent L36 A2
  constraint tangent L35 A2
  constraint tangent L35 A3
  constraint tangent L34 A3
  measures "d138" radius of A0
  measures "d139" radius of A1
  measures "d140" radius of A2
  measures "d141" radius of A3
extrude "Extrude6'" add sketch "Sketch7" along normal blind 169.8625 contours L0 L1 L2 L3 L12 L22 | E0 L4 L5 E1 L6 E2 L7 E3 L34 L35 L36 L37 A0 A1 A2 A3 picked at (-33.455761, 29.36875) picked at (-8.329698, -32.808333) bodies 2 3 4 5 6 7 in component "enclosure"
sketch "Sketch8 (2)" plane through (0, 171.45, 0) normal (0, 1, 0) x (-1, 0, 0) in component "enclosure"
  line L0 (71.4375, -28.575) -> (-71.4375, -28.575)
  line L1 (-71.4375, -28.575) -> (-71.4375, 28.575)
  line L2 (-71.4375, 28.575) -> (71.4375, 28.575)
  line L3 (71.4375, 28.575) -> (71.4375, -28.575)
  arc A0 (73.2155, -34.925) -> (77.7875, -30.353) centre (73.2155, -30.353) ccw
  line L4 (77.7875, -30.353) -> (77.7875, 30.353)
  arc A1 (77.7875, 30.353) -> (73.2155, 34.925) centre (73.2155, 30.353) ccw
  line L5 (73.2155, 34.925) -> (-73.2155, 34.925)
  arc A2 (-73.2155, 34.925) -> (-77.7875, 30.353) centre (-73.2155, 30.353) ccw
  line L6 (-77.7875, 30.353) -> (-77.7875, -30.353)
  arc A3 (-77.7875, -30.353) -> (-73.2155, -34.925) centre (-73.2155, -30.353) ccw
  line L7 (-73.2155, -34.925) -> (73.2155, -34.925)
  line L8 (73.2155, 34.925) -> (-73.2155, 34.925)
  arc A4 (-73.2155, 34.925) -> (-77.7875, 30.353) centre (-73.2155, 30.353) ccw
  line L9 (-77.7875, 30.353) -> (-77.7875, -30.353)
  arc A5 (-77.7875, -30.353) -> (-73.2155, -34.925) centre (-73.2155, -30.353) ccw
  line L10 (-73.2155, -34.925) -> (73.2155, -34.925)
  arc A6 (73.2155, -34.925) -> (77.7875, -30.353) centre (73.2155, -30.353) ccw
  line L11 (77.7875, -30.353) -> (77.7875, 30.353)
  arc A7 (77.7875, 30.353) -> (73.2155, 34.925) centre (73.2155, 30.353) ccw
  line L12 (-75.40625, 30.353) -> (-75.40625, -30.353)
  arc A8 (-75.40625, -30.353) -> (-73.2155, -32.54375) centre (-73.2155, -30.353) ccw
  line L13 (-73.2155, -32.54375) -> (73.2155, -32.54375)
  arc A9 (73.2155, -32.54375) -> (75.40625, -30.353) centre (73.2155, -30.353) ccw
  line L14 (75.40625, -30.353) -> (75.40625, 30.353)
  arc A10 (75.40625, 30.353) -> (73.2155, 32.54375) centre (73.2155, 30.353) ccw
  line L15 (73.2155, 32.54375) -> (-73.2155, 32.54375)
  arc A11 (-73.2155, 32.54375) -> (-75.40625, 30.353) centre (-73.2155, 30.353) ccw
  line L16 (-71.4375, 28.575) -> (71.4375, 28.575)
  line L17 (-71.4375, -28.575) -> (-71.4375, 28.575)
  line L18 (71.4375, -28.575) -> (-71.4375, -28.575)
  line L19 (71.4375, 28.575) -> (71.4375, -28.575)
extrude "Extrude7'" cut sketch "Sketch8 (2)" against normal up to surface (157.1625 mm away) contours L12 A8 L13 A9 L14 A10 L15 A11 picked at (23.8125, -31.220833) bodies 2 in component "enclosure"
sketch "Sketch10 (2)" plane through (0, 0, 0) normal (1, 0, 0) x (0, 1, 0) in component "enclosure"
  line L0 (14.2875, 28.575) -> (14.2875, -28.575)
  line L1 (14.2875, -28.575) -> (14.2875, 28.575)
  line L2 (14.2875, 30.353) -> (14.2875, -30.353)
  line L3 (14.2875, -32.54375) -> (14.2875, -30.353)
  line L4 (14.2875, -32.54375) -> (14.2875, -30.353)
  line L5 (14.2875, -30.353) -> (14.2875, 30.353)
  line L6 (14.2875, 30.353) -> (14.2875, 32.54375)
  line L7 (14.2875, 30.353) -> (14.2875, 32.54375)
  line L8 (14.2875, -32.54375) -> (171.45, -32.54375)
  line L9 (171.45, -32.54375) -> (14.2875, -32.54375)
  line L10 (14.2875, -28.575) -> (14.2875, -32.54375)
  line L11 (14.2875, -32.54375) -> (18.25625, -32.54375)
  line L12 (14.2875, -28.575) -> (18.25625, -32.54375)
  constraint coincident L0.end L1.start
  constraint perpendicular L3 L11
  constraint equal L10 L11
sweep "Sweep1'" add profiles "Sketch10 (2)" along 8 edges at (-75.40625, 14.2875, 0) (-74.764594, 14.2875, 31.902094) (0, 14.2875, 32.54375) (74.764594, 14.2875, 31.902094) (75.40625, 14.2875, 0) (74.764594, 14.2875, -31.902094) (0, 14.2875, -32.54375) (-74.764594, 14.2875, -31.902094) section 1 on bodies 2 bodies 2 in component "enclosure"